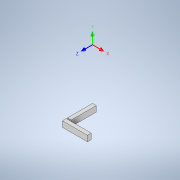
# Autodesk Inventor part: 2edificios
Saved by Autodesk Inventor 2021 (Build 250183000, 183)
## iProperties
Created: 2021-06-17
Part Number: 2edificios
Material: Genérico
Document SubType Name: Modeling
Designer: luise
Density: 1 g/cm^3
Appearance: Valor por defecto
Author: luise
Autodesk Inventor part; units mm, degrees
ref_plane "YZ Plane" through (0, 0, 0) normal (1, 0, 0) x (0, 1, 0)
ref_plane "XZ Plane" through (0, 0, 0) normal (0, 1, 0) x (-1, 0, 0)
ref_plane "XY Plane" through (0, 0, 0) normal (0, 0, 1) x (1, 0, 0)
sketch "Boceto1" plane through (0, 0, 0) normal (0, 1, 0) x (-1, 0, 0)
  line L0 (-180000, 276000) -> (-260000, 276000)
  line L1 (-260000, 276000) -> (-260000, 264000)
  line L2 (-260000, 264000) -> (-180000, 264000)
  line L3 (-180000, 264000) -> (-180000, 276000)
  line L4 (-180000, 260000) -> (-192000, 260000)
  line L5 (-192000, 260000) -> (-192000, 180000)
  line L6 (-192000, 180000) -> (-180000, 180000)
  line L7 (-180000, 180000) -> (-180000, 260000)
  line L8 (-548000, 0) -> (0, 0)
  line L9 (0, 0) -> (0, 456000)
  line L10 (-548000, 456000) -> (-548000, 0)
  line L11 (-548000, 456000) -> (0, 456000)
  point P0 (0, 0)
  dimension "d0" = 80000
  dimension "d1" = 12000
  dimension "d2" = 12000
  dimension "d3" = 80000
  dimension "d13" = 180000
  dimension "d14" = 288000
  dimension "d15" = 548000
  dimension "d17" = 4000
  dimension "d19" = 180000
  dimension "d20" = 180000
  dimension "d21" = 456000
  constraints: 24 end point, 5 parallel, 3 horizontal, 3 perpendicular
  measures "d0" distance of L2.end L1.end
  measures "d1" distance of L1.end L0.end
  measures "d2" distance of L6.end L5.end
  measures "d3" distance of L5.end L4.end
  measures "d13" distance between parallel lines of L9 L7
  measures "d14" distance between parallel lines of L1 L10
  measures "d15" distance between parallel lines of L9 L10
  measures "d17" distance between parallel lines of L2 L4
  measures "d19" distance between parallel lines of L11 L0
  measures "d20" distance between parallel lines of L8 L6
  measures "d21" distance between parallel lines of L11 L8
extrude "Extrusión1" add sketch "Boceto1" along normal blind 18000 contours L3 L2 L1 L0 | L7 L6 L5 L4
sketch "Boceto2" plane through (0, 0, 0) normal (0, 1, 0) x (-1, 0, 0)
  line L0 (0, 0) -> (0, 456000) projected
  line L1 (-548000, 456000) -> (0, 456000) projected
  line L2 (-548000, 456000) -> (-548000, 0) projected
  line L3 (-548000, 0) -> (0, 0) projected
  point P0 (0, 0)
  dimension "d24" = 548000
  dimension "d25" = 456000
  measures "d24" distance between parallel lines of L0 L2
  measures "d25" distance between parallel lines of L1 L3
extrude "Extrusión2" [suppressed]
